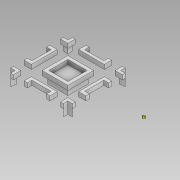
# Autodesk Inventor part: CrossRail-DSS
Saved by Autodesk Inventor 2021 (Build 250183000, 183)
## iProperties
Created: 2021-05-27
Part Number: CrossRail-DSS
Material: 一般
Document SubType Name: Modeling
Designer: kumagai
Density: 1 g/cm^3
Appearance: 既定
Author: kumagai
Autodesk Inventor part; units mm, degrees
ref_plane "YZ Plane" through (0, 0, 0) normal (1, 0, 0) x (0, 1, 0)
ref_plane "XZ Plane" through (0, 0, 0) normal (0, 1, 0) x (-1, 0, 0)
ref_plane "XY Plane" through (0, 0, 0) normal (0, 0, 1) x (1, 0, 0)
sketch "スケッチ1" plane through (0, 0, 0) normal (0, 1, 0) x (-1, 0, 0)
  line L0 (0, -64.5) -> (0, 10.75) projected
  line L1 (-64.5, 0) -> (10.75, 0) projected
  line L2 (0, 0) -> (0, -22.264)
  line L3 (0, -22.264) -> (-19, -22.264)
  line L4 (-19, -22.264) -> (-19, -19)
  line L5 (-19, -19) -> (-22.264, -19)
  line L6 (-22.264, -19) -> (-22.264, 0)
  line L7 (-22.264, 0) -> (0, 0)
  line L8 (-17, -22.264) -> (-17, -17)
  line L9 (-17, -17) -> (-22.264, -17)
  line L10 (-9.3, -22.264) -> (-9.3, -17)
  line L11 (-9.3, -17) -> (0, -17)
  line L12 (0, -19) -> (-6.9, -19)
  line L13 (-6.9, -19) -> (-6.9, -22.264)
  line L14 (-22.264, -9.3) -> (-17, -9.3)
  line L15 (-17, -9.3) -> (-17, 0)
  line L16 (-19, 0) -> (-19, -6.9)
  line L17 (-19, -6.9) -> (-22.264, -6.9)
  line L18 (0, -6.9) -> (-6.9, -6.9)
  line L19 (-6.9, -6.9) -> (-6.9, 0)
  line L20 (0, -9.3) -> (-9.3, -9.3)
  line L21 (-9.3, -9.3) -> (-9.3, 0)
  dimension "d0" = 19
  dimension "d1" = 19
  dimension "d2" = 22.264
  dimension "d3" = 22.264
  dimension "d4" = 9.3
  dimension "d5" = 2.4
  dimension "d6" = 2
  dimension "d7" = 2
  dimension "d8" = 9.3
  dimension "d9" = 2.4
  constraints: 40 end point, 20 point on line, 9 vertical, 7 horizontal, 6 collinear
  measures "d0" distance between parallel lines of L4 L2
  measures "d1" distance between parallel lines of L7 L5
  measures "d2" distance between parallel lines of L1 L3
  measures "d3" distance between parallel lines of L2 L6
  measures "d4" distance between parallel lines of L2 L10
  measures "d5" distance between parallel lines of L10 L13
  measures "d6" distance between parallel lines of L4 L8
  measures "d7" distance between parallel lines of L9 L5
  measures "d8" distance between parallel lines of L7 L14
  measures "d9" distance between parallel lines of L14 L17
extrude "押し出し1" add sketch "スケッチ1" along normal blind 3.2 contours L12 L13 L3 L10 L11 L0 | L20 L21 L1 L19 L18 L0 | L3 L4 L5 L6 L9 L8 | L15 L14 L6 L17 L16 L1
extrude "押し出し2" add sketch "スケッチ1" against normal blind 5.2
sketch "スケッチ2" plane through (0, 0, 0) normal (0, 1, 0) x (-1, 0, 0)
  line L0 (0, -22.264) -> (-19, -22.264) projected
  line L1 (-17, -22.264) -> (-17, -17) projected
  line L2 (-22.264, -19) -> (-22.264, 0) projected
  line L3 (-17, -17) -> (-22.264, -17) projected
  line L4 (0, -64.5) -> (0, 10.75) projected
  line L5 (-64.5, 0) -> (10.75, 0) projected
  line L6 (-19, -22.264) -> (-17, -7.264)
  line L7 (-17, -7.264) -> (0, -7.264)
  line L8 (-22.264, -19) -> (-7.264, -17)
  line L9 (-7.264, -17) -> (-7.264, 0)
  line L10 (0, -22.264) -> (0, -7.264)
  line L11 (-7.264, 0) -> (-22.264, 0)
  point P0 (0, 0)
  dimension "d16" = 15
  dimension "d17" = 15
  constraints: 12 end point, 4 point on line, 2 horizontal, 2 vertical
  measures "d16" distance between parallel lines of L0 L7
  measures "d17" distance between parallel lines of L2 L9
extrude "押し出し3" cut sketch "スケッチ2" against normal through all contours L0 L1 L8 L9 L7 L4 | L0 L6 L8 L1 | L8 L6 L3 L1 | L1 L3 L6 L7 L9 L8 | L7 L6 L3 L2 L5 L9 | L8 L2 L3 L6
mirror "ミラー1" about plane through (0, 0, 0) normal (1, 0, 0) of "押し出し1", "押し出し2", "押し出し3"
mirror "ミラー2" about plane through (0, 0, 0) normal (0, 0, 1) of "押し出し1", "押し出し2", "押し出し3", "ミラー1"
equation "\"d0\" = 0.5 * RailWidth"
equation "\"d1\" = 0.5 * RailWidth"
equation "\"d2\" = 0.5 * LengthB"
equation "\"d3\" = 0.5 * LengthA"
equation "\"d4\" = 0.5 * InsideWidth"
equation "\"d5\" = InnerWall"
equation "\"d6\" = OuterWall"
equation "\"d7\" = OuterWall"
equation "\"d8\" = 0.5 * InsideWidth"
equation "\"d9\" = InnerWall"
equation "\"d12\" = RailDepth"
equation "\"d14\" = RailHeight - RailDepth"
equation "\"LengthA\" = 0.207107 * StraightLength"
equation "\"LengthB\" = LengthA"
equation "\"RailWidth\" = 38"
equation "\"InsideWidth\" = 18.6"
equation "\"InnerWall\" = 2.4"
equation "\"OuterWall\" = 2"
equation "\"RailDepth\" = 3.2"
equation "\"RailHeight\" = 8.4"
equation "\"StraightLength\" = 215"
